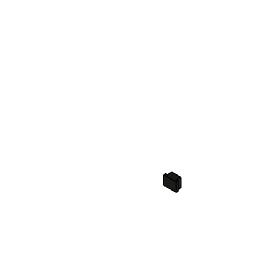
Taste_links_v56 (Autodesk Fusion 360 design; units mm, degrees)
Autodesk Fusion 360 part; units mm, degrees
sketch "Skizze1" plane through (0, 0, 59.536) normal (0, 0, -1) x (1, 0, 0)
  line L0 (54.288, -85.97) -> (62.288, -85.97)
  line L1 (62.288, -85.97) -> (62.288, -82.97)
  line L2 (62.288, -82.97) -> (54.288, -82.97)
  line L3 (54.288, -82.97) -> (54.288, -85.97)
  line L4 (63.688, -82.82) -> (62.188, -82.82)
  line L5 (62.188, -82.82) -> (62.188, -86.47)
  line L6 (62.188, -86.47) -> (54.588, -86.47)
  line L7 (54.588, -86.47) -> (54.588, -82.82)
  line L8 (54.588, -82.82) -> (53.088, -82.82)
  line L9 (53.088, -82.82) -> (53.088, -81.07)
  line L10 (53.088, -81.07) -> (63.688, -81.07)
  line L11 (63.688, -81.07) -> (63.688, -82.82)
  line L12 (50.288, -82.97) -> (50.288, -85.97)
  line L13 (56.538, -80.97) -> (60.038, -80.97)
  line L14 (40.65, -82.97) -> (67.1, -82.97)
  line L15 (-54.35, -82.97) -> (27.15, -82.97)
  point P0 (54.288, -85.97)
  point P1 (50.288, -85.97)
  dimension "d139_1_2_4" = 1.5
  dimension "d140_1_2_4" = 1.5
  dimension "d1144" = 7.6
  dimension "d1145" = 1.75
  dimension "d1146" = 3.65
  constraint horizontal L4
  constraint perpendicular L0 L5
  constraint perpendicular L5 L6
  constraint perpendicular L0 L7
  constraint perpendicular L7 L8
  constraint perpendicular L0 L9
  constraint perpendicular L7 L10
  constraint perpendicular L10 L11
  constraint horizontal L4.end L7.end
  measures "d139_1_2_4" distance of L7.end L8.end
  measures "d140_1_2_4" distance of L4.start L4.end
  measures "d1144" distance of L5.end L6.end
  measures "d1145" distance of L8.end L9.end
  measures "d1146" distance of L6.end L7.end
extrude "Extrusion1" add sketch "Skizze1" along normal blind 7.6 contours L0 L2 L5 L7 L14 | L0 L5 L6 L7 | L2 L4 L5 L7 L8 L9 L10 L11 L14
sketch "Skizze2" plane through (0, 86.47, 0) normal (0, 1, 0) x (-1, 0, 0)
  line L0 (-54.588, 59.536) -> (-62.188, 59.536)
  line L1 (-62.188, 59.536) -> (-62.188, 51.936)
  line L2 (-62.188, 51.936) -> (-54.588, 51.936)
  line L3 (-54.588, 51.936) -> (-54.588, 59.536)
  line L4 (-55.288, 56.486) -> (-58.288, 56.486)
  line L5 (-58.288, 56.486) -> (-58.288, 58.036)
  line L6 (-58.288, 58.036) -> (-61.488, 55.736)
  line L7 (-61.488, 55.736) -> (-58.288, 53.436)
  line L8 (-58.288, 53.436) -> (-58.288, 54.986)
  line L9 (-58.288, 54.986) -> (-55.288, 54.986)
  line L10 (-55.288, 54.986) -> (-55.288, 56.486)
  point P0 (-62.188, 55.736)
  point P1 (-55.288, 55.736)
  dimension "d385" = 0.7
  dimension "d386" = 0.7
  dimension "d387" = 1.5
  dimension "d388" = 1.5
  dimension "d389" = 1.5
  dimension "d390" = 3
  constraint horizontal L4
  constraint perpendicular L4 L5
  constraint parallel L5 L8
  constraint perpendicular L8 L9
  constraint perpendicular L9 L10
  constraint midpoint L1 P0
  constraint vertical L4.end L8.end
  constraint horizontal L6.end P0
  constraint midpoint L10 P1
  constraint horizontal P0 P1
  measures "d385" distance of L3 L10
  measures "d386" distance of L1 L6.end
  measures "d387" distance of L0 L5.end
  measures "d388" distance of L2 L7.end
  measures "d389" distance of L4 L9
  measures "d390" distance of L4.start L4.end
emboss "Prägen1" depth 1 profiles "Skizze2" section 1 contours L4 L5 L6 L7 L8 L9 L10 onto face at (59.6547, 86.47, 54.4693)
move_body "Verschieben1" bodies 1 to x (1, 0, 0) y (0, 1, 0) z (0, 0, 1) at (36, 0, -35.8)
equation "d140_1_2_4 = d139_1_2_4"
equation "d388 = d387"
